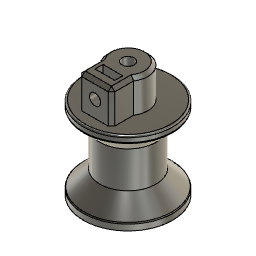
enrouleur_porte_poule_v0-0-5 v2 (Autodesk Fusion 360 design; units mm, degrees)
Autodesk Fusion 360 part; units mm, degrees
note: some values were not read from the file. Chosen so that the rebuilt part matches the saved one: which face or edge a step refers to; which pieces of a blend or face edit are solid.
sketch "Esquisse1" plane through (0, 0, 0) normal (0, 0, 1) x (1, 0, 0)
  circle A0 centre (0, 0) radius 1.85
  circle A1 centre (0, 0) radius 8.5
  circle A2 centre (0, 0) radius 13.5
  dimension "d1" = 3.7
  dimension "d2" = 17
  dimension "d3" = 27
  constraint coincident A0.centre A1.centre
  constraint concentric A0 A2
  measures "d1" diameter of A0
  measures "d2" diameter of A1
  measures "d3" diameter of A2
extrude "Extrusion1" add sketch "Esquisse1" along normal blind 25 contours A1
ref_plane "Plan de construction1" through (0, 0, 12.5) normal (0, 0, 1) x (1, 0, 0)
extrude "Extrusion2" add sketch "Esquisse1" along normal blind 2 contours A2
chamfer "Chanfrein1" distance 5 angle 45 1 edges at (-7.9248, -3.0737, 2)
mirror "Symétrie miroir1" about plane through (0, 0, 12.5) normal (0, 0, 1) of "Extrusion2", "Chanfrein1"
sketch "Esquisse2" plane through (0, 0, 25) normal (0, 0, 1) x (-1, 0, 0)
  circle A0 centre (0, 0) radius 13.5
  circle A1 centre (0, 0) radius 1.85
  circle A2 centre (0, 0) radius 6
  line L0 (0, 0) -> (5, 0)
  line L1 (5, 0) -> (5, 10)
  line L2 (5, 10) -> (0, 10)
  line L3 (0, 10) -> (0, 0)
  line L4 (-5, 0) -> (-5, 10)
  line L5 (0, 0) -> (-5, 0)
  line L6 (-5, 10) -> (0, 10)
  dimension "d12" = 12
  dimension "d15" = 5
  dimension "d16" = 10
  constraint coincident A0.centre A1.centre
  constraint horizontal L0
  constraint vertical L1
  constraint horizontal L2
  constraint vertical L3
  constraint symmetric A0.centre L3 A1.centre
  constraint symmetric L0.end L3 L4.start
  constraint symmetric L1.end L3 L4.end
  constraint symmetric L2.end L3 L6.end
  measures "d12" diameter of A2
  measures "d15" distance of A0.centre L0.end
  measures "d16" distance of A0.centre L2.end
extrude "Extrusion3" add sketch "Esquisse2" along normal blind 10 contours A1 A2 L0 L1 L4 L5 | A1 A2 L0 L1 L3 | A1 A2 L3 L4 L5 | A2 L1 L2 L3 | A2 L3 L4 L6
ref_plane "Plan de construction2" through (0, -7, 30) normal (0, -1, 0) x (1, 0, 0)
sketch "Esquisse3" plane through (0, -7, 0) normal (0, -1, 0) x (1, 0, 0)
  line L0 (-5, 25) -> (5, 25)
  line L1 (5, 25) -> (5, 35)
  line L2 (-5, 35) -> (-5, 25)
  line L3 (0, 35) -> (0, 25) construction
  line L4 (0, 35) -> (-3, 35)
  line L5 (-3, 35) -> (-3, 30)
  line L6 (-3, 30) -> (0, 30) construction
  line L7 (-3, 30) -> (-3, 28.27)
  line L8 (-3, 28.27) -> (0, 26.3)
  line L9 (3, 30) -> (0, 30) construction
  line L10 (3, 35) -> (3, 30)
  line L11 (3, 30) -> (3, 28.27)
  line L12 (3, 28.27) -> (0, 26.3)
  line L13 (0, 35) -> (3, 35)
  dimension "d28" = 1.73
  dimension "d29" = 3.7
  dimension "d30" = 3
  dimension "d31" = 5
  constraint midpoint L0 L3.end
  constraint perpendicular L0 L3
  constraint perpendicular L3 L4
  constraint perpendicular L4 L5
  constraint coincident L3 L6.end
  constraint perpendicular L3 L6
  constraint perpendicular L6 L7
  constraint coincident L3 L8.end
  constraint symmetric L4.start L3 L13.start
  constraint symmetric L3 L4.end L10.start
  constraint symmetric L3 L5.end L9.start
  constraint symmetric L3 L6.end L9.end
  constraint symmetric L3 L7.end L11.end
  constraint symmetric L3 L8.end L12.end
  measures "d28" distance of L5.end L7.end
  measures "d29" distance of L6 L8.end
  measures "d30" distance of L3 L5
  measures "d31" distance of L4.end L5.end
sketch "Esquisse4" plane through (0, -10, 0) normal (0, -1, 0) x (1, 0, 0)
  circle A0 centre (0, 30) radius 1.7
  line L0 (-5, 25) -> (5, 25)
  line L1 (5, 25) -> (5, 35)
  line L2 (5, 35) -> (-5, 35)
  line L3 (-5, 35) -> (-5, 25)
  point P0 (0, 30)
  dimension "d22" = 3.4
  constraint coincident P0 A0.centre
  measures "d22" diameter of A0
extrude "Extrusion5" cut sketch "Esquisse4" against normal blind 10 contours A0
extrude "Extrusion6" cut sketch "Esquisse3" against normal blind 2.4
chamfer "Chanfrein2" distance 1 angle 45 6 edges at (5, -6.6583, 35) (0, 6, 35) (-5, -6.6583, 35) (0, -10, 35) (5, -10, 30) (-5, -10, 30)
fillet "Congé1" radius 0.5 1 edges at (-12.5864, -4.8818, 25)
fillet "Congé2" radius 0.5 4 edges at (-13.5, 0, 23) (-13.499, 0, 23) (-13.499, 0, 2) (-13.5, 0, 2)
chamfer "Chanfrein3" distance 1 angle 45 1 edges at (-1.7248, 0.669, 0)
equation "d4 = 25 mm"
equation "d6 = -d4 / 2"
